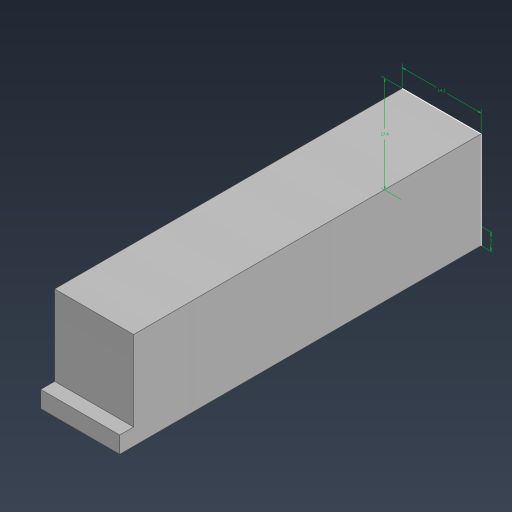
# Autodesk Inventor part: tattu450_2s
Saved by Autodesk Inventor 2023 (Build 270158000, 158)
## iProperties
Created: 2024-10-28
Part Number: tattu450_2s
Material: Ogólny
Document SubType Name: Sheet Metal
Designer: krako
Density: 2.70716 g/cm^3
Sheet Metal Rule: Default_mm
Appearance: Jasnoszara
Mass: 37 g
Surface Area: 40.4695 cm^2
Volume: 13.6674 cm^3
Author: krako
Autodesk Inventor part; units mm, degrees
ref_plane "YZ Plane" through (0, 0, 0) normal (1, 0, 0) x (0, 1, 0)
ref_plane "XZ Plane" through (0, 0, 0) normal (0, 1, 0) x (-1, 0, 0)
ref_plane "XY Plane" through (0, 0, 0) normal (0, 0, 1) x (1, 0, 0)
sketch "Szkic1" plane through (0, 0, 0) normal (0, 0, 1) x (1, 0, 0)
  line L0 (0, 0) -> (-14.2, 0)
  line L1 (-14.2, 0) -> (-14.2, 17.4)
  line L2 (-14.2, 17.4) -> (0, 17.4)
  line L3 (0, 17.4) -> (0, 0)
  line L4 (-14.2, 3) -> (0, 3)
  dimension "d0" = 14.2
  dimension "d1" = 17.4
  dimension "d8" = 3
  constraints: 10 end point, 2 parallel, 2 perpendicular, 2 point on line, 1 horizontal
  measures "d0" distance of L1.end L2.end
  measures "d1" distance of L0.end L1.end
  measures "d8" distance between parallel lines of L0 L4
extrude "Extrusion2" add sketch "Szkic1" along normal blind 62.5
extrude "Extrusion3" add sketch "Szkic1" along normal blind 65 contours L0 L1 L4 L3
equation "\"PromieńGięcia\" = Grubość"
equation "\"SzerokośćGięciaPodcięcia\" = Grubość"
equation "\"GłębokośćGięciaPodcięcia\" = 0.5 * Grubość"
equation "\"RozmiarPodcięciaNarożnika\" = 4 * Grubość"
equation "\"MinimalnaPozostałość\" = 2 * Grubość"
equation "\"PromieńPrzejścia\" = PromieńGięcia"
equation "\"Rozmiar_promienia_Jacobiego\" = PromieńGięcia"
equation "\"Wielk_odstępu\" = Grubość"
equation "\"Grubość\" = 0.5"
body "Solid2"
